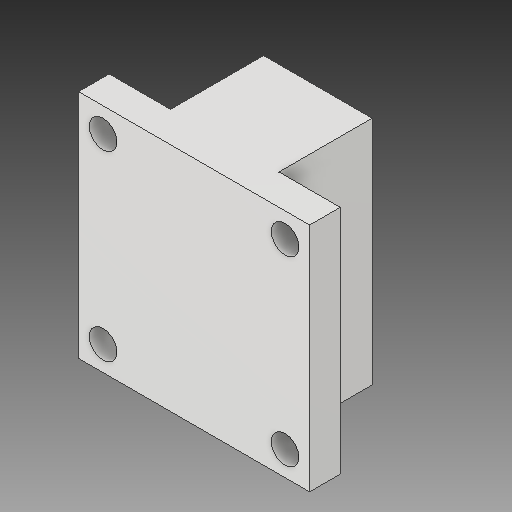
# Autodesk Inventor part: CornerBracket
Saved by Autodesk Inventor 2019.3 (Build 233278000, 278)
## iProperties
Created: 2019-06-25
Part Number: CornerBracket
Material: PC/ABS Plastic
Document SubType Name: Modeling
Designer: mark
Density: 0.357273 g/cm^3
Appearance: Smooth - White
Author: mark
Autodesk Inventor part; units mm, degrees
ref_plane "YZ Plane" through (0, 0, 0) normal (1, 0, 0) x (0, 1, 0)
ref_plane "XZ Plane" through (0, 0, 0) normal (0, 1, 0) x (-1, 0, 0)
ref_plane "XY Plane" through (0, 0, 0) normal (0, 0, 1) x (1, 0, 0)
sketch "Sketch1" plane through (0, 0, 0) normal (0, 0, 1) x (1, 0, 0)
  line L0 (0, 0) -> (25.4, 0) projected
  line L1 (25.4, 0) -> (25.4, 500) projected
  line L2 (0, 500) -> (25.4, 500) projected
  line L3 (0, 0) -> (0, 500) projected
  line L4 (115.4, 0) -> (140.8, 0) projected
  line L5 (140.8, 0) -> (140.8, 500) projected
  line L6 (115.4, 500) -> (140.8, 500) projected
  line L7 (115.4, 0) -> (115.4, 500) projected
  line L8 (-25, 505) -> (50.4, 505)
  line L9 (50.4, 505) -> (50.4, 429.6)
  line L10 (50.4, 429.6) -> (-25, 429.6)
  line L11 (-25, 429.6) -> (-25, 505)
  circle A0 centre (-17, 437.6) radius 4.5
  circle A1 centre (-17, 497) radius 4.5
  circle A2 centre (42.4, 497) radius 4.5
  circle A3 centre (42.4, 437.6) radius 4.5
  dimension "d0" = 25
  dimension "d31" = 25
  dimension "d32" = 5
  dimension "d33" = 9
  dimension "d34" = 9
  dimension "d35" = 9
  dimension "d36" = 9
  dimension "d37" = 8
  dimension "d38" = 8
  dimension "d39" = 8
  dimension "d40" = 8
  dimension "d41" = 8
  dimension "d42" = 8
  dimension "d43" = 8
  dimension "d44" = 8
  constraints: 8 end point, 4 centre point, 1 horizontal, 1 parallel, 1 perpendicular
  measures "d0" distance between parallel lines of L3 L11
  measures "d31" distance between parallel lines of L1 L9
  measures "d32" distance between parallel lines of L8 L2
  measures "d33" diameter of A1
  measures "d34" diameter of A0
  measures "d35" diameter of A2
  measures "d36" diameter of A3
  measures "d37" distance from line of L8 A1.centre
  measures "d38" distance from line of L11 A1.centre
  measures "d39" distance from line of A0.centre L11
  measures "d40" distance from line of A0.centre L10
  measures "d41" distance from line of L9 A3.centre
  measures "d42" distance from line of A3.centre L10
  measures "d43" distance from line of L9 A2.centre
  measures "d44" distance from line of L8 A2.centre
extrude "Extrusion1" add sketch "Sketch1" along normal blind 10 contours L10 L11 L8 L9 L1 L2 L3 | L3 L2 L1 L10
sketch "Sketch3" plane through (0, 0, 0) normal (0, 0, -1) x (-1, 0, 0)
  line L0 (5, 505) -> (-30.4, 505)
  line L1 (-30.4, 505) -> (-30.4, 500)
  line L2 (-30.4, 500) -> (5, 500)
  line L3 (5, 500) -> (5, 505)
  line L4 (25, 505) -> (-50.4, 505) projected
  line L5 (25, 429.6) -> (25, 505) projected
  point P0 (0, 0)
  dimension "d45" = 35.4
  dimension "d46" = 20
  dimension "d47" = 5
  constraints: 8 end point, 1 collinear
  measures "d45" distance between parallel lines of L1 L3
  measures "d46" distance between parallel lines of L5 L3
  measures "d47" distance between parallel lines of L0 L2
extrude "Extrusion2" add sketch "Sketch3" along normal blind 30.4
sketch "Sketch5" plane through (-5, 500, 0) normal (0, -1, 0) x (1, 0, 0)
  line L0 (0, -30.4) -> (5, -30.4)
  line L1 (5, -30.4) -> (5, 0)
  line L2 (5, 0) -> (0, 0)
  line L3 (0, 0) -> (0, -30.4)
  line L4 (5, -30.4) -> (30.4, -30.4)
  line L5 (30.4, -30.4) -> (30.4, -25.4)
  line L6 (30.4, -25.4) -> (5, -25.4)
  line L7 (5, -25.4) -> (5, -30.4)
  line L8 (35.4, -30.4) -> (30.4, -30.4)
  line L9 (30.4, -30.4) -> (30.4, 0)
  line L10 (30.4, 0) -> (35.4, 0)
  line L11 (35.4, 0) -> (35.4, -30.4)
  line L12 (55.4, 0) -> (-20, 0) projected
  line L13 (35.4, -30.4) -> (0, -30.4) projected
  line L14 (0, 0) -> (0, -30.4) projected
  line L15 (35.4, 0) -> (35.4, -30.4) projected
  point P0 (5, 0)
  dimension "d48" = 5
  dimension "d49" = 25.4
  dimension "d50" = 25.4
  constraints: 24 end point, 9 collinear, 1 point on line
  measures "d48" distance between parallel lines of L3 L1
  measures "d49" distance between parallel lines of L6 L12
  measures "d50" distance between parallel lines of L1 L9
extrude "Extrusion4" add sketch "Sketch5" along normal up to surface (70.4 mm away) contours L3 L2 L1 L0 | L1 L6 L5 L4 | L5 L9 L10 L11 L8
body "Solid1"
